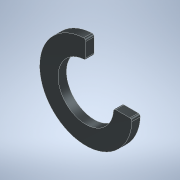
# Autodesk Inventor part: 503.017.01_Splint_Feder
Saved by Autodesk Inventor 2021 (Build 250183000, 183)
## iProperties
Created: 2021-11-23
Part Number: 503.017.01_Splint_Feder
Material: Eisen, Grau
Document SubType Name: Modeling
Designer: Sebastian Seewald
Mass: 1.25844 g
Surface Area: 3.30924 cm^2
Volume: 0.176005 cm^3
Density: 7.15 g/cm^3
Appearance: Eisen - Grau
Author: Sebastian Seewald
Autodesk Inventor part; units mm, degrees
ref_plane "YZ Plane" through (0, 0, 0) normal (1, 0, 0) x (0, 1, 0)
ref_plane "XZ Plane" through (0, 0, 0) normal (0, 1, 0) x (-1, 0, 0)
ref_plane "XY Plane" through (0, 0, 0) normal (0, 0, 1) x (1, 0, 0)
sketch "Skizze1" plane through (0, 0, 0) normal (0, 0, 1) x (1, 0, 0)
  circle A0 centre (0, 0) radius 11
  circle A1 centre (0, 0) radius 6.6
  line L0 (0, 11) -> (0, 6.6)
  line L1 (11, 0) -> (6.6, 0)
  dimension "d0" = 13.2
  dimension "d1" = 22
  constraints: 4 end point, 4 point on circle, 2 centre point, 2 coincident, 1 perpendicular, 1 vertical
  measures "d0" diameter of A1
  measures "d1" diameter of A0
extrude "Extrusion1" add sketch "Skizze1" along normal blind 2 contours A0 L0 A1 L1 picked at (9.3538, -1.4402)
fillet "Rundung1" radius 0.5 4 edges at (0, 11, 1) (0, 6.6, 1) (6.6, 0, 1) (11, 0, 1)
